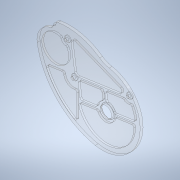
# Autodesk Inventor part: 足外フレーム
Saved by Autodesk Inventor 2022.2 (Build 262287010, 287A)
## iProperties
Created: 2022-01-10
Part Number: 足外フレーム
Material: Polycarbonate, Clear
Document SubType Name: Modeling
Designer: acps
Density: 1.2 g/cm^3
Appearance: Polycarbonate - Clear
Author: acps
Autodesk Inventor part; units mm, degrees
ref_plane "YZ Plane" through (0, 0, 0) normal (1, 0, 0) x (0, 1, 0)
ref_plane "XZ Plane" through (0, 0, 0) normal (0, 1, 0) x (-1, 0, 0)
ref_plane "XY Plane" through (0, 0, 0) normal (0, 0, 1) x (1, 0, 0)
sketch "Sketch6" plane through (0, 0, 0) normal (0, 0, 1) x (1, 0, 0)
  circle A0 centre (46.616, 30) radius 14 construction
  circle A1 centre (67.0906, 21) radius 20.5 construction
  circle A2 centre (100, 0) radius 30 construction
  arc A3 (42.888, 47.6097) -> (28.8489, 27.1141) centre (46.616, 30) ccw
  arc A4 (89.1412, -35.261) -> (103.4815, 41.4054) centre (96.6972, 3) ccw
  arc A5 (28.8489, 27.1141) -> (89.1412, -35.261) centre (103.8658, 39.2989) ccw
  line L0 (-13.9923, -60) -> (152.4896, -60) construction
  arc A6 (128.8918, 13.9322) -> (111.061, 33.8169) centre (96.6972, 3) ccw construction
  circle A7 centre (122.6202, 25) radius 3
  circle A8 centre (58.1571, 43.8132) radius 3
  circle A9 centre (65.359, 13) radius 3
  circle A10 centre (58.1571, 43.8132) radius 4 construction
  arc A11 (42.888, 47.6097) -> (45.3636, 50.3845) centre (42.2376, 50.6816) ccw
  arc A12 (50.502, 55.8582) -> (45.3636, 50.3845) centre (51.4661, 49.8045) ccw
  arc A13 (93.5981, 45.5879) -> (50.502, 55.8582) centre (59.6238, -1.42) ccw
  arc A14 (93.5981, 45.5879) -> (103.4815, 41.4054) centre (107.6564, 65.0395) ccw
  line L1 (78.7064, -36) -> (126.3698, -36) construction
  circle A15 centre (58.1571, 43.8132) radius 1.5
  circle A16 centre (65.359, 13) radius 1.5
  circle A17 centre (100, 0) radius 6.025
  circle A18 centre (122.6202, 25) radius 1.5
  arc A19 (68.1719, 47.9001) -> (64.0942, 44.6795) centre (67.0628, 45.1126) ccw
  line L2 (64.0942, 44.6795) -> (67.7217, 19.8179)
  arc A20 (67.7217, 19.8179) -> (71.1234, 17.2824) centre (70.6903, 20.251) ccw
  arc A21 (114.185, 23.5655) -> (114.8611, 29.3215) centre (113.7519, 26.5341) ccw
  line L3 (71.1234, 17.2824) -> (114.185, 23.5655)
  circle A22 centre (122.6202, 25) radius 6 construction
  circle A23 centre (58.1571, 43.8132) radius 6 construction
  circle A24 centre (65.359, 13) radius 6 construction
  line L4 (68.1719, 47.9001) -> (114.8611, 29.3215)
  line L5 (73.0578, 14.5329) -> (93.8988, 17.5738)
  arc A25 (96.1666, 15.8835) -> (93.8988, 17.5738) centre (94.1875, 15.5947) ccw
  line L6 (96.1666, 15.8835) -> (97.0063, 10.1286)
  arc A26 (95.9293, 8.0548) -> (97.0063, 10.1286) centre (95.0272, 9.8398) ccw
  arc A27 (95.9293, 8.0548) -> (91.1178, 1.5994) centre (100, 0) ccw
  arc A28 (89.4383, -0.0252) -> (91.1178, 1.5994) centre (89.1495, 1.9539) ccw
  line L7 (75.4791, -2.0619) -> (89.4383, -0.0252)
  line L8 (100, 0) -> (96.9289, 21.0477) construction
  arc A29 (73.0578, 14.5329) -> (71.3675, 12.2651) centre (73.3465, 12.5539) ccw
  line L9 (71.3675, 12.2651) -> (73.2113, -0.3716)
  arc A30 (73.2113, -0.3716) -> (75.4791, -2.0619) centre (75.1903, -0.0829) ccw
  line L10 (129.6856, 4.3314) -> (73.0213, -3.9364) construction
  arc A31 (100.8254, 18.5844) -> (99.1351, 16.3166) centre (101.1142, 16.6054) ccw
  line L11 (99.1351, 16.3166) -> (99.9748, 10.5617)
  arc A32 (99.9748, 10.5617) -> (101.5994, 8.8821) centre (101.9539, 10.8505) ccw
  line L12 (100.8254, 18.5844) -> (117.068, 20.9544)
  arc A33 (118.6726, 20.4815) -> (117.068, 20.9544) centre (117.3568, 18.9753) ccw
  arc A34 (108.0548, 4.0707) -> (101.5994, 8.8821) centre (100, 0) ccw
  arc A35 (108.0548, 4.0707) -> (110.1286, 2.9937) centre (109.8398, 4.9728) ccw
  line L13 (110.1286, 2.9937) -> (128.6428, 5.6951)
  arc A36 (128.6428, 5.6951) -> (130.3326, 7.9663) centre (128.354, 7.6742) ccw
  arc A37 (118.6726, 20.4815) -> (124.5936, 19.3338) centre (122.6202, 25) ccw
  arc A38 (127.036, 18.3479) -> (124.5936, 19.3338) centre (125.2514, 17.4451) ccw
  arc A39 (130.3326, 7.9663) -> (127.036, 18.3479) centre (96.6972, 3) ccw
  arc A40 (91.9452, -4.0707) -> (108.8821, -1.5994) centre (100, 0) ccw
  arc A41 (91.9452, -4.0707) -> (89.8714, -2.9937) centre (90.1602, -4.9728) ccw
  arc A42 (110.5617, 0.0252) -> (108.8821, -1.5994) centre (110.8505, -1.9539) ccw
  line L14 (110.5617, 0.0252) -> (126.7332, 2.3847)
  line L15 (89.8714, -2.9937) -> (73.6999, -5.3533)
  arc A43 (73.6999, -5.3533) -> (72.0637, -7.875) centre (73.9887, -7.3323) ccw
  arc A44 (129.0217, 0.4357) -> (126.7332, 2.3847) centre (127.0219, 0.4057) ccw
  arc A45 (72.0637, -7.875) -> (129.0217, 0.4357) centre (100, 0) ccw
  arc A46 (51.2056, 43.2263) -> (58.8155, 36.8682) centre (46.616, 30) ccw
  arc A47 (52.4518, 41.9559) -> (51.2056, 43.2263) centre (50.55, 41.3368) ccw
  arc A48 (58.8155, 36.8682) -> (57.3438, 37.8686) centre (57.0728, 35.887) ccw
  arc A49 (52.4518, 41.9559) -> (57.3438, 37.8686) centre (58.1571, 43.8132) ccw
  arc A50 (38.5312, 9.0435) -> (67.0636, -22.5849) centre (103.8658, 39.2989) ccw
  arc A51 (40.0572, 11.863) -> (38.5312, 9.0435) centre (40.346, 9.884) ccw
  line L16 (40.0572, 11.863) -> (54.1218, 13.9151)
  arc A52 (56.4012, 12.1295) -> (54.1218, 13.9151) centre (54.4105, 11.9361) ccw
  arc A53 (56.4012, 12.1295) -> (67.5901, 4.2809) centre (65.359, 13) ccw
  arc A54 (70.0859, 2.3434) -> (67.5901, 4.2809) centre (68.0859, 2.3434) ccw
  line L17 (70.0859, 2.3434) -> (70.0859, -20.8659)
  arc A55 (67.0636, -22.5849) -> (70.0859, -20.8659) centre (68.0859, -20.8659) ccw
  arc A56 (34.4673, 18.1085) -> (59.1679, 18.5348) centre (46.616, 30) ccw construction
  circle A57 centre (100, 0) radius 7
  point P0 (0, 0)
  point P1 (0, 0)
  point P2 (100, 0)
  point P3 (44.5807, 48.5912)
  point P4 (46.9968, 54)
  point P5 (73.0693, 55)
  dimension "d116" = 4
  dimension "d117" = 60
  dimension "d118" = 76
  dimension "d119" = 39
  dimension "d120" = 5
  dimension "d121" = 6
  dimension "d122" = 6
  dimension "d123" = 25
  dimension "d124" = 6
  dimension "d125" = 37
  dimension "d126" = 13
  dimension "d127" = 1
  dimension "d128" = 3.14
  dimension "d129" = 6.13
  dimension "d130" = 58
  dimension "d131" = 24
  dimension "d132" = 48.5912
  dimension "d133" = 54
  dimension "d134" = 55
  dimension "d135" = 42.888
  dimension "d136" = 24
  dimension "d137" = 3
  dimension "d138" = 3
  dimension "d139" = 12.05
  dimension "d140" = 3
  dimension "d141" = 3
  dimension "d142" = 3
  dimension "d143" = 3
  dimension "d144" = 3
  dimension "d145" = 3
  dimension "d146" = 3
  dimension "d147" = 30
  dimension "d148" = 90
  dimension "d149" = 2
  dimension "d150" = 2
  dimension "d151" = 3
  dimension "d152" = 2
  dimension "d153" = 2
  dimension "d154" = 2
  dimension "d155" = 3
  dimension "d156" = 1.5
  dimension "d157" = 1.5
  dimension "d158" = 2
  dimension "d159" = 2
  dimension "d160" = 2
  dimension "d161" = 3
  dimension "d162" = 1.5
  dimension "d163" = 3
  dimension "d164" = 2
  dimension "d165" = 1.5
  dimension "d166" = 2
  dimension "d167" = 2
  dimension "d168" = 2
  dimension "d169" = 2
  dimension "d170" = 3
  dimension "d171" = 1.5
  dimension "d172" = 1.5
  dimension "d173" = 2
  dimension "d174" = 2
  dimension "d175" = 20
  dimension "d176" = 2
  dimension "d177" = 2
  dimension "d178" = 2
  dimension "d179" = 4
  constraints: 95 point on circle, 66 tangent, 57 centre point, 36 end point, 13 concentric, 10 parallel, 5 coincident, 2 horizontal, 2 perpendicular, 2 point on line, 1 vertical, 7 other
  measures "d116" radial gap between concentric circles of A0 A3
  measures "d117" distance from line of L0 point (0, 0)
  measures "d118" radius of A5
  measures "d119" radius of A4
  measures "d120" radial gap between concentric circles of A4 A6
  measures "d121" diameter of A7
  measures "d122" diameter of A8
  measures "d123" vertical distance of point (0, 0) A7.centre
  measures "d124" diameter of A9
  measures "d125" distance of point (100, 0) A9.centre
  measures "d126" vertical distance of point (0, 0) A9.centre
  measures "d127" radial gap between concentric circles of A8 A10
  measures "d128" radius of A11
  measures "d129" radius of A12
  measures "d130" radius of A13
  measures "d131" radius of A14
  measures "d132" vertical distance of point (0, 0) point (44.581, 48.591)
  measures "d133" vertical distance of point (0, 0) point (46.997, 54)
  measures "d134" vertical distance of point (0, 0) point (73.069, 55)
  measures "d135" horizontal distance of point (0, 0) A3.start
  measures "d136" distance between parallel lines of L0 L1
  measures "d137" diameter of A15
  measures "d138" diameter of A16
  measures "d139" diameter of A17
  measures "d140" diameter of A18
  measures "d141" radius of A19
  measures "d142" radius of A20
  measures "d143" radius of A21
  measures "d144" radial gap between concentric circles of A7 A22
  measures "d145" radial gap between concentric circles of A8 A23
  measures "d146" radial gap between concentric circles of A9 A24
  measures "d147" angle of L3 L4
  measures "d148" angle of L3 L2
  measures "d149" radius of A25
  measures "d150" radius of A26
  measures "d151" radial gap between concentric circles of A17 A27
  measures "d152" radius of A28
  measures "d153" radius of A29
  measures "d154" radius of A30
  measures "d155" distance between parallel lines of L3 L5
  measures "d156" distance between parallel lines of L8 L6
  measures "d157" distance between parallel lines of L10 L7
  measures "d158" radius of A31
  measures "d159" radius of A32
  measures "d160" radius of A33
  measures "d161" distance between parallel lines of L12 L3
  measures "d162" distance between parallel lines of L8 L11
  measures "d163" radial gap between concentric circles of A17 A34
  measures "d164" radius of A35
  measures "d165" distance between parallel lines of L10 L13
  measures "d166" radius of A36
  measures "d167" radius of A38
  measures "d168" radius of A41
  measures "d169" radius of A42
  measures "d170" radial gap between concentric circles of A40 A17
  measures "d171" distance between parallel lines of L15 L10
  measures "d172" distance between parallel lines of L10 L14
  measures "d173" radius of A43
  measures "d174" radius of A44
  measures "d175" radial gap between concentric circles of A45 A40
  measures "d176" radius of A47
  measures "d177" radius of A48
  measures "d178" radius of A51
  measures "d179" radial gap between concentric circles of A5 A50
extrude "Extrusion4" add sketch "Sketch6" along normal blind 3 contours A11 A12 A13 A14 A4 A5 A3 | A57
extrude "Extrusion5" add sketch "Sketch6" along normal blind 1 contours L4 A21 L3 A20 L2 A19 | L5 A25 L6 A26 A27 A28 L7 A30 L9 A29 | L12 A33 A37 A38 A39 A36 L13 A35 A34 A32 L11 A31 | A40 A42 L14 A44 A45 A43 L15 A41 | A51 L16 A52 A53 A54 L17 A55 A50
sketch "Sketch7" plane through (0, 0, 3) normal (0, 0, 1) x (1, 0, 0)
  circle A0 centre (58.1571, 43.8132) radius 3 projected
  circle A1 centre (58.1571, 43.8132) radius 1.5 projected
  circle A2 centre (65.359, 13) radius 3 projected
  circle A3 centre (65.359, 13) radius 1.5 projected
  circle A4 centre (122.6202, 25) radius 3 projected
  circle A5 centre (122.6202, 25) radius 1.5 projected
  point P0 (0, 0)
extrude "Extrusion6" add sketch "Sketch7" against normal blind 2
extrude "Extrusion7" cut sketch "Sketch6" along normal blind 1 contours A57
sketch "Sketch8" plane through (0, 0, 3) normal (0, 0, 1) x (1, 0, 0)
  arc A0 (51.2056, 43.2263) -> (58.8155, 36.8682) centre (46.616, 30) ccw projected
  arc A1 (52.4518, 41.9559) -> (57.3438, 37.8686) centre (58.1571, 43.8132) ccw projected
  arc A2 (52.4518, 41.9559) -> (51.2056, 43.2263) centre (50.55, 41.3368) ccw projected
  arc A3 (58.8155, 36.8682) -> (57.3438, 37.8686) centre (57.0728, 35.887) ccw projected
  point P0 (0, 0)
extrude "Extrusion8" add sketch "Sketch8" against normal blind 1
body "Solid2"
